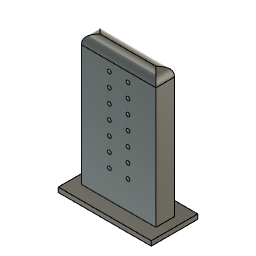
Camera_Stand (Autodesk Fusion 360 design; units mm, degrees)
Autodesk Fusion 360 part; units mm, degrees
sketch "Sketch1" plane through (0, 0, 0) normal (0, 0, 1) x (1, 0, 0) in component "base"
  line L0 (-50, -25) -> (50, -25)
  line L1 (50, -25) -> (50, 25)
  line L2 (50, 25) -> (-50, 25)
  line L3 (-50, 25) -> (-50, -25)
  constraint horizontal L0
  constraint vertical L1
  constraint horizontal L2
  constraint vertical L3
extrude "Extrude1" add sketch "Sketch1" along normal blind 5 makes body 1 in component "base"
sketch "Sketch1 (2)" plane through (0, 0, 5) normal (0, 0, 1) x (-1, 0, 0) in component "Component"
  line L0 (50, -25) -> (50, 25)
  line L1 (50, 25) -> (-50, 25)
  line L2 (-50, 25) -> (-50, -25)
  line L3 (-50, -25) -> (50, -25)
  line L4 (40, -10) -> (-40, -10)
  line L5 (-40, -10) -> (-40, 10)
  line L6 (-40, 10) -> (40, 10)
  line L7 (40, 10) -> (40, -10)
  dimension "d3" = 80
  constraint horizontal L4
  constraint vertical L5
  constraint horizontal L6
  constraint vertical L7
  measures "d3" distance of L4.start L4.end
extrude "Extrude1'" add sketch "Sketch1 (2)" along normal blind 140 separate body contours L4 L5 L6 L7 makes body 2 in component "Component"
sketch "Sketch2" plane through (0, -10, 0) normal (0, -1, 0) x (1, 0, 0) in component "Component"
  line L0 (-40, 5) -> (40, 5)
  line L1 (40, 5) -> (40, 145)
  line L2 (40, 145) -> (-40, 145)
  line L3 (-40, 145) -> (-40, 5)
sketch "Sketch1 (3)" plane through (0, -10, 0) normal (0, -1, 0) x (1, 0, 0) in component "holes"
  circle A0 centre (-10, 125) radius 2
  circle A1 centre (10, 125) radius 2
  circle A2 centre (-10, 110) radius 2
  circle A3 centre (10, 110) radius 2
  circle A4 centre (-10, 95) radius 2
  circle A5 centre (10, 95) radius 2
  circle A6 centre (-10, 80) radius 2
  circle A7 centre (10, 80) radius 2
  circle A8 centre (-10, 65) radius 2
  circle A9 centre (10, 65) radius 2
  circle A10 centre (-10, 50) radius 2
  circle A11 centre (10, 50) radius 2
  circle A12 centre (-10, 35) radius 2
  circle A13 centre (10, 35) radius 2
  dimension "d7" = 4
  dimension "d8" = 4
  dimension "d9" = 4
  dimension "d10" = 4
  dimension "d11" = 4
  dimension "d12" = 4
  dimension "d13" = 4
  dimension "d14" = 4
  dimension "d15" = 4
  dimension "d16" = 4
  dimension "d17" = 4
  dimension "d18" = 4
  dimension "d19" = 4
  dimension "d20" = 4
  measures "d7" diameter of A0
  measures "d8" diameter of A1
  measures "d9" diameter of A2
  measures "d10" diameter of A3
  measures "d11" diameter of A4
  measures "d12" diameter of A5
  measures "d13" diameter of A6
  measures "d14" diameter of A7
  measures "d15" diameter of A8
  measures "d16" diameter of A9
  measures "d17" diameter of A10
  measures "d18" diameter of A11
  measures "d19" diameter of A12
  measures "d20" diameter of A13
hole "Hole1" at (-10, -10, 125) at (10, -10, 125) at (-10, -10, 110) at (10, -10, 110) at (10, -10, 95) at (-10, -10, 95) at (-10, -10, 80) at (10, -10, 80) at (10, -10, 65) at (-10, -10, 65) at (-10, -10, 50) at (10, -10, 50) at (10, -10, 35) at (-10, -10, 35) direction (0, 1, 0) diameter 4 depth 45 tip angle 118 bodies 2 in component "Component"
fillet "Fillet1" radius 10 tangency weight 1.47804 1 faces at (-13.3333, 3.3333, 145) on bodies 2 in component "Component"
component "base" placed x (1, 0, 0) y (0, 1, 0) z (0, 0, 1) at (0, 0, 0)
component "Component" placed x (1, 0, 0) y (0, 1, 0) z (0, 0, 1) at (0, 0, 0)
component "holes" placed x (1, 0, 0) y (0, 1, 0) z (0, 0, 1) at (0, 0, 0)
